Autodesk Fusion 360 part; units mm, degrees
(part 3 of 3)
  line L0 (23, 43.2567) -> (0, 43.2567)
  line L1 (0, 43.2567) -> (0, 32.1215)
  line L2 (0, 32.1215) -> (23, 32.1215)
  line L3 (23, 32.1215) -> (23, 43.2567)
  point P0 (22.9203, 43.2088)
  point P1 (22.8408, 43.161)
  point P2 (22.7615, 43.1132)
  point P3 (22.6824, 43.0656)
  point P4 (22.6036, 43.018)
  point P5 (22.5249, 42.9705)
  point P6 (22.4465, 42.9231)
  point P7 (22.3683, 42.8757)
  point P8 (22.2903, 42.8285)
  point P9 (22.2126, 42.7813)
  point P10 (22.135, 42.7342)
  point P11 (22.0577, 42.6872)
  point P12 (21.9806, 42.6403)
  point P13 (21.9036, 42.5935)
  point P14 (21.827, 42.5468)
  point P15 (21.7505, 42.5001)
  point P16 (21.6742, 42.4536)
  point P17 (21.5981, 42.4071)
  point P18 (21.5223, 42.3607)
  point P19 (21.4467, 42.3144)
  point P20 (21.3713, 42.2682)
  point P21 (21.2961, 42.2221)
  point P22 (21.2211, 42.1761)
  point P23 (21.1463, 42.1302)
  point P24 (21.0717, 42.0844)
  point P25 (20.9973, 42.0386)
  point P26 (20.9232, 41.993)
  point P27 (20.8492, 41.9475)
  point P28 (20.7755, 41.902)
  point P29 (20.702, 41.8567)
  point P30 (20.6287, 41.8115)
  point P31 (20.5556, 41.7663)
  point P32 (20.4827, 41.7213)
  point P33 (20.41, 41.6763)
  point P34 (20.3375, 41.6315)
  point P35 (20.2652, 41.5867)
  point P36 (20.1931, 41.5421)
  point P37 (20.1212, 41.4975)
  point P38 (20.0496, 41.4531)
  point P39 (19.9781, 41.4087)
  point P40 (19.9068, 41.3645)
  point P41 (19.8358, 41.3204)
  point P42 (19.7649, 41.2763)
  point P43 (19.6943, 41.2324)
  point P44 (19.6238, 41.1886)
  point P45 (19.5536, 41.1448)
  point P46 (19.4835, 41.1012)
  point P47 (19.4137, 41.0577)
  point P48 (19.344, 41.0143)
  point P49 (19.2746, 40.971)
  point P50 (19.2054, 40.9278)
  point P51 (19.1363, 40.8848)
  point P52 (19.0674, 40.8418)
  point P53 (18.9988, 40.7989)
  point P54 (18.9303, 40.7562)
  point P55 (18.8621, 40.7135)
  point P56 (18.794, 40.671)
  point P57 (18.7261, 40.6285)
  point P58 (18.6585, 40.5862)
  point P59 (18.591, 40.544)
  point P60 (18.5237, 40.5019)
  point P61 (18.4566, 40.4599)
  point P62 (18.3897, 40.418)
  point P63 (18.323, 40.3763)
  point P64 (18.2565, 40.3346)
  point P65 (18.1901, 40.2931)
  point P66 (18.124, 40.2516)
  point P67 (18.0581, 40.2103)
  point P68 (17.9923, 40.1691)
  point P69 (17.9267, 40.128)
  point P70 (17.8613, 40.0871)
  point P71 (17.7962, 40.0462)
  point P72 (17.7311, 40.0054)
  point P73 (17.6663, 39.9648)
  point P74 (17.6017, 39.9243)
  point P75 (17.5373, 39.8839)
  point P76 (17.473, 39.8436)
  point P77 (17.4089, 39.8034)
  point P78 (17.345, 39.7633)
  point P79 (17.2813, 39.7234)
  point P80 (17.2178, 39.6835)
  point P81 (17.1544, 39.6438)
  point P82 (17.0913, 39.6042)
  point P83 (17.0283, 39.5647)
  point P84 (16.9655, 39.5254)
  point P85 (16.9029, 39.4861)
  point P86 (16.8404, 39.447)
  point P87 (16.7781, 39.408)
  point P88 (16.7161, 39.3691)
  point P89 (16.6541, 39.3303)
  point P90 (16.5924, 39.2916)
  point P91 (16.5309, 39.2531)
  point P92 (16.4695, 39.2146)
  point P93 (16.4083, 39.1763)
  point P94 (16.3472, 39.1381)
  point P95 (16.2864, 39.1)
  point P96 (16.2257, 39.0621)
  point P97 (16.1652, 39.0242)
  point P98 (16.1048, 38.9865)
  point P99 (16.0447, 38.9489)
  point P100 (15.9847, 38.9114)
  point P101 (15.9248, 38.874)
  point P102 (15.8652, 38.8368)
  point P103 (15.8057, 38.7997)
  point P104 (15.7464, 38.7626)
  point P105 (15.6872, 38.7257)
  point P106 (15.6282, 38.689)
  point P107 (15.5694, 38.6523)
  point P108 (15.5107, 38.6158)
  point P109 (15.4522, 38.5793)
  point P110 (15.3939, 38.543)
  point P111 (15.3357, 38.5068)
  point P112 (15.2778, 38.4708)
  point P113 (15.2199, 38.4348)
  point P114 (15.1622, 38.399)
  point P115 (15.1047, 38.3633)
  point P116 (15.0474, 38.3277)
  point P117 (14.9902, 38.2922)
  point P118 (14.9332, 38.2569)
  point P119 (14.8763, 38.2216)
  point P120 (14.8196, 38.1865)
  point P121 (14.763, 38.1515)
  point P122 (14.7066, 38.1167)
  point P123 (14.6504, 38.0819)
  point P124 (14.5943, 38.0473)
  point P125 (14.5384, 38.0127)
  point P126 (14.4826, 37.9783)
  point P127 (14.427, 37.9441)
  point P128 (14.3715, 37.9099)
  point P129 (14.3162, 37.8758)
  point P130 (14.261, 37.8419)
  point P131 (14.206, 37.8081)
  point P132 (14.1511, 37.7744)
  point P133 (14.0964, 37.7408)
  point P134 (14.0419, 37.7074)
  point P135 (13.9875, 37.6741)
  point P136 (13.9332, 37.6408)
  point P137 (13.8791, 37.6077)
  point P138 (13.8251, 37.5748)
  point P139 (13.7713, 37.5419)
  point P140 (13.7176, 37.5092)
  point P141 (13.6641, 37.4765)
  point P142 (13.6107, 37.444)
  point P143 (13.5575, 37.4116)
  point P144 (13.5044, 37.3794)
  point P145 (13.4514, 37.3472)
  point P146 (13.3986, 37.3152)
  point P147 (13.3459, 37.2832)
  point P148 (13.2934, 37.2514)
  point P149 (13.241, 37.2198)
  point P150 (13.1888, 37.1882)
  point P151 (13.1367, 37.1567)
  point P152 (13.0847, 37.1254)
  point P153 (13.0329, 37.0942)
  point P154 (12.9812, 37.0631)
  point P155 (12.9296, 37.0321)
  point P156 (12.8782, 37.0012)
  point P157 (12.8269, 36.9705)
  point P158 (12.7758, 36.9398)
  point P159 (12.7248, 36.9093)
  point P160 (12.6739, 36.8789)
  point P161 (12.6232, 36.8486)
  point P162 (12.5725, 36.8184)
  point P163 (12.5221, 36.7884)
  point P164 (12.4717, 36.7584)
  point P165 (12.4215, 36.7286)
  point P166 (12.3714, 36.6989)
  point P167 (12.3215, 36.6693)
  point P168 (12.2716, 36.6398)
  point P169 (12.2219, 36.6104)
  point P170 (12.1724, 36.5812)
  point P171 (12.1229, 36.5521)
  point P172 (12.0736, 36.523)
  point P173 (12.0244, 36.4941)
  point P174 (11.9753, 36.4653)
  point P175 (11.9264, 36.4366)
  point P176 (11.8776, 36.4081)
  point P177 (11.8289, 36.3796)
  point P178 (11.7803, 36.3513)
  point P179 (11.7319, 36.323)
  point P180 (11.6836, 36.2949)
  point P181 (11.6354, 36.2669)
  point P182 (11.5873, 36.239)
  point P183 (11.5393, 36.2112)
  point P184 (11.4915, 36.1836)
  point P185 (11.4438, 36.156)
  point P186 (11.3962, 36.1286)
  point P187 (11.3487, 36.1012)
  point P188 (11.3013, 36.074)
  point P189 (11.2541, 36.0469)
  point P190 (11.2069, 36.0199)
  point P191 (11.1599, 35.993)
  point P192 (11.113, 35.9662)
  point P193 (11.0662, 35.9396)
  point P194 (11.0196, 35.913)
  point P195 (10.973, 35.8866)
  point P196 (10.9265, 35.8602)
  point P197 (10.8802, 35.834)
  point P198 (10.834, 35.8079)
  point P199 (10.7879, 35.7819)
  point P200 (10.7419, 35.756)
  point P201 (10.696, 35.7302)
  point P202 (10.6502, 35.7045)
  point P203 (10.6046, 35.6789)
  point P204 (10.559, 35.6535)
  point P205 (10.5135, 35.6281)
  point P206 (10.4682, 35.6028)
  point P207 (10.423, 35.5777)
  point P208 (10.3778, 35.5527)
  point P209 (10.3328, 35.5277)
  point P210 (10.2879, 35.5029)
  point P211 (10.2431, 35.4782)
  point P212 (10.1984, 35.4536)
  point P213 (10.1538, 35.4291)
  point P214 (10.1093, 35.4047)
  point P215 (10.0649, 35.3804)
  point P216 (10.0206, 35.3563)
  point P217 (9.9764, 35.3322)
  point P218 (9.9323, 35.3082)
  point P219 (9.8883, 35.2844)
  point P220 (9.8444, 35.2606)
  point P221 (9.8006, 35.2369)
  point P222 (9.7569, 35.2134)
  point P223 (9.7133, 35.19)
  point P224 (9.6698, 35.1666)
  point P225 (9.6264, 35.1434)
  point P226 (9.5831, 35.1202)
  point P227 (9.5399, 35.0972)
  point P228 (9.4968, 35.0743)
  point P229 (9.4538, 35.0515)
  point P230 (9.4109, 35.0288)
  point P231 (9.3681, 35.0061)
  point P232 (9.3253, 34.9836)
  point P233 (9.2827, 34.9612)
  point P234 (9.2402, 34.9389)
  point P235 (9.1977, 34.9167)
  point P236 (9.1553, 34.8946)
  point P237 (9.1131, 34.8726)
  point P238 (9.0709, 34.8507)
  point P239 (9.0288, 34.8289)
  point P240 (8.9868, 34.8072)
  point P241 (8.9449, 34.7856)
  point P242 (8.9031, 34.7641)
  point P243 (8.8614, 34.7427)
  point P244 (8.8197, 34.7214)
  point P245 (8.7782, 34.7002)
  point P246 (8.7367, 34.6791)
  point P247 (8.6953, 34.6581)
  point P248 (8.6541, 34.6373)
  point P249 (8.6128, 34.6165)
  point P250 (8.5717, 34.5958)
  point P251 (8.5307, 34.5752)
  point P252 (8.4897, 34.5547)
  point P253 (8.4489, 34.5343)
  point P254 (8.4081, 34.514)
  point P255 (8.3674, 34.4937)
  point P256 (8.3268, 34.4736)
  point P257 (8.2862, 34.4536)
  point P258 (8.2458, 34.4337)
  point P259 (8.2054, 34.4139)
  point P260 (8.1651, 34.3942)
  point P261 (8.1249, 34.3746)
  point P262 (8.0848, 34.355)
  point P263 (8.0447, 34.3356)
  point P264 (8.0048, 34.3163)
  point P265 (7.9649, 34.297)
  point P266 (7.925, 34.2779)
  point P267 (7.8853, 34.2588)
  point P268 (7.8456, 34.2399)
  point P269 (7.806, 34.221)
  point P270 (7.7665, 34.2023)
  point P271 (7.7271, 34.1836)
  point P272 (7.6877, 34.165)
  point P273 (7.6485, 34.1466)
  point P274 (7.6093, 34.1282)
  point P275 (7.5701, 34.1099)
  point P276 (7.5311, 34.0917)
  point P277 (7.4921, 34.0736)
  point P278 (7.4531, 34.0556)
  point P279 (7.4143, 34.0377)
  point P280 (7.3755, 34.0198)
  point P281 (7.3368, 34.0021)
  point P282 (7.2982, 33.9845)
  point P283 (7.2596, 33.9669)
  point P284 (7.2211, 33.9495)
  point P285 (7.1827, 33.9321)
  point P286 (7.1444, 33.9148)
  point P287 (7.1061, 33.8977)
  point P288 (7.0679, 33.8806)
  point P289 (7.0297, 33.8636)
  point P290 (6.9917, 33.8467)
  point P291 (6.9536, 33.8299)
  point P292 (6.9157, 33.8131)
  point P293 (6.8778, 33.7965)
  point P294 (6.84, 33.78)
  point P295 (6.8023, 33.7635)
  point P296 (6.7646, 33.7472)
  point P297 (6.727, 33.7309)
  point P298 (6.6894, 33.7147)
  point P299 (6.6519, 33.6986)
  point P300 (6.6145, 33.6826)
  point P301 (6.5771, 33.6667)
  point P302 (6.5398, 33.6509)
  point P303 (6.5026, 33.6351)
  point P304 (6.4654, 33.6195)
  point P305 (6.4283, 33.6039)
  point P306 (6.3913, 33.5885)
  point P307 (6.3543, 33.5731)
  point P308 (6.3173, 33.5578)
  point P309 (6.2805, 33.5426)
  point P310 (6.2437, 33.5274)
  point P311 (6.2069, 33.5124)
  point P312 (6.1702, 33.4975)
  point P313 (6.1336, 33.4826)
  point P314 (6.097, 33.4678)
  point P315 (6.0605, 33.4532)
  point P316 (6.024, 33.4386)
  point P317 (5.9876, 33.424)
  point P318 (5.9513, 33.4096)
  point P319 (5.915, 33.3953)
  point P320 (5.8788, 33.381)
  point P321 (5.8426, 33.3669)
  point P322 (5.8064, 33.3528)
  point P323 (5.7704, 33.3388)
  point P324 (5.7344, 33.3249)
  point P325 (5.6984, 33.311)
  point P326 (5.6625, 33.2973)
  point P327 (5.6266, 33.2837)
  point P328 (5.5908, 33.2701)
  point P329 (5.5551, 33.2566)
  point P330 (5.5194, 33.2432)
  point P331 (5.4837, 33.2299)
  point P332 (5.4481, 33.2166)
  point P333 (5.4126, 33.2035)
  point P334 (5.3771, 33.1904)
  point P335 (5.3417, 33.1774)
  point P336 (5.3063, 33.1645)
  point P337 (5.2709, 33.1517)
  point P338 (5.2356, 33.139)
  point P339 (5.2004, 33.1263)
  point P340 (5.1652, 33.1138)
  point P341 (5.13, 33.1013)
  point P342 (5.0949, 33.0889)
  point P343 (5.0599, 33.0766)
  point P344 (5.0249, 33.0643)
  point P345 (4.9899, 33.0522)
  point P346 (4.955, 33.0401)
  point P347 (4.9201, 33.0281)
  point P348 (4.8853, 33.0162)
  point P349 (4.8505, 33.0044)
  point P350 (4.8158, 32.9927)
  point P351 (4.7811, 32.981)
  point P352 (4.7465, 32.9694)
  point P353 (4.7119, 32.9579)
  point P354 (4.6773, 32.9465)
  point P355 (4.6428, 32.9352)
  point P356 (4.6084, 32.9239)
  point P357 (4.5739, 32.9127)
  point P358 (4.5396, 32.9016)
  point P359 (4.5052, 32.8906)
  point P360 (4.4709, 32.8797)
  point P361 (4.4367, 32.8689)
  point P362 (4.4025, 32.8581)
  point P363 (4.3683, 32.8474)
  point P364 (4.3341, 32.8368)
  point P365 (4.3001, 32.8262)
  point P366 (4.266, 32.8158)
  point P367 (4.232, 32.8054)
  point P368 (4.198, 32.7951)
  point P369 (4.1641, 32.7849)
  point P370 (4.1302, 32.7748)
  point P371 (4.0963, 32.7647)
  point P372 (4.0625, 32.7548)
  point P373 (4.0287, 32.7449)
  point P374 (3.995, 32.7351)
  point P375 (3.9612, 32.7253)
  point P376 (3.9276, 32.7157)
  point P377 (3.8939, 32.7061)
  point P378 (3.8603, 32.6966)
  point P379 (3.8268, 32.6872)
  point P380 (3.7932, 32.6778)
  point P381 (3.7597, 32.6686)
  point P382 (3.7263, 32.6594)
  point P383 (3.6928, 32.6503)
  point P384 (3.6595, 32.6413)
  point P385 (3.6261, 32.6323)
  point P386 (3.5928, 32.6235)
  point P387 (3.5595, 32.6147)
  point P388 (3.5262, 32.6059)
  point P389 (3.493, 32.5973)
  point P390 (3.4598, 32.5888)
  point P391 (3.4266, 32.5803)
  point P392 (3.3935, 32.5719)
  point P393 (3.3604, 32.5636)
  point P394 (3.3273, 32.5553)
  point P395 (3.2943, 32.5471)
  point P396 (3.2613, 32.5391)
  point P397 (3.2283, 32.531)
  point P398 (3.1954, 32.5231)
  point P399 (3.1624, 32.5152)
  point P400 (3.1295, 32.5075)
  point P401 (3.0967, 32.4998)
  point P402 (3.0638, 32.4921)
  point P403 (3.031, 32.4846)
  point P404 (2.9983, 32.4771)
  point P405 (2.9655, 32.4697)
  point P406 (2.9328, 32.4624)
  point P407 (2.9001, 32.4552)
  point P408 (2.8674, 32.448)
  point P409 (2.8348, 32.4409)
  point P410 (2.8022, 32.4339)
  point P411 (2.7696, 32.427)
  point P412 (2.737, 32.4202)
  point P413 (2.7045, 32.4134)
  point P414 (2.672, 32.4067)
  point P415 (2.6395, 32.4001)
  point P416 (2.607, 32.3935)
  point P417 (2.5746, 32.387)
  point P418 (2.5421, 32.3807)
  point P419 (2.5098, 32.3743)
  point P420 (2.4774, 32.3681)
  point P421 (2.445, 32.3619)
  point P422 (2.4127, 32.3559)
  point P423 (2.3804, 32.3499)
  point P424 (2.3481, 32.3439)
  point P425 (2.3159, 32.3381)
  point P426 (2.2836, 32.3323)
  point P427 (2.2514, 32.3266)
  point P428 (2.2192, 32.321)
  point P429 (2.187, 32.3154)
  point P430 (2.1549, 32.31)
  point P431 (2.1227, 32.3046)
  point P432 (2.0906, 32.2993)
  point P433 (2.0585, 32.294)
  point P434 (2.0265, 32.2889)
  point P435 (1.9944, 32.2838)
  point P436 (1.9624, 32.2788)
  point P437 (1.9303, 32.2739)
  point P438 (1.8983, 32.269)
  point P439 (1.8663, 32.2642)
  point P440 (1.8344, 32.2595)
  point P441 (1.8024, 32.2549)
  point P442 (1.7705, 32.2504)
  point P443 (1.7386, 32.2459)
  point P444 (1.7067, 32.2415)
  point P445 (1.6748, 32.2372)
  point P446 (1.6429, 32.233)
  point P447 (1.6111, 32.2288)
  point P448 (1.5792, 32.2248)
  point P449 (1.5474, 32.2208)
  point P450 (1.5156, 32.2168)
  point P451 (1.4838, 32.213)
  point P452 (1.452, 32.2092)
  point P453 (1.4202, 32.2055)
  point P454 (1.3885, 32.2019)
  point P455 (1.3567, 32.1984)
  point P456 (1.325, 32.1949)
  point P457 (1.2933, 32.1916)
  point P458 (1.2616, 32.1883)
  point P459 (1.2299, 32.185)
  point P460 (1.1982, 32.1819)
  point P461 (1.1665, 32.1788)
  point P462 (1.1349, 32.1758)
  point P463 (1.1032, 32.1729)
  point P464 (1.0716, 32.1701)
  point P465 (1.04, 32.1674)
  point P466 (1.0083, 32.1647)
  point P467 (0.9767, 32.1621)
  point P468 (0.9451, 32.1596)
  point P469 (0.9135, 32.1571)
  point P470 (0.882, 32.1548)
  point P471 (0.8504, 32.1525)
  point P472 (0.8188, 32.1503)
  point P473 (0.7873, 32.1482)
  point P474 (0.7557, 32.1462)
  point P475 (0.7242, 32.1442)
  point P476 (0.6926, 32.1423)
  point P477 (0.6611, 32.1405)
  point P478 (0.6296, 32.1388)
  point P479 (0.5981, 32.1372)
  point P480 (0.5666, 32.1356)
  point P481 (0.535, 32.1341)
  point P482 (0.5035, 32.1327)
  point P483 (0.472, 32.1314)
  point P484 (0.4406, 32.1302)
  point P485 (0.4091, 32.129)
  point P486 (0.3776, 32.128)
  point P487 (0.3461, 32.127)
  point P488 (0.3146, 32.1261)
  point P489 (0.2832, 32.1253)
  point P490 (0.2517, 32.1245)
  point P491 (0.2202, 32.1238)
  point P492 (0.1888, 32.1233)
  point P493 (0.1573, 32.1228)
  point P494 (0.1258, 32.1223)
  point P495 (0.0944, 32.122)
  point P496 (0.0629, 32.1218)
  point P497 (0.0315, 32.1216)
  constraint horizontal L0
  constraint vertical L1
  constraint horizontal L2
  constraint vertical L3
revolve "回転1" add sketch "スケッチ1" angle 360 about axis through (0, 43.2567, 0) along (0, -1, 0) contours S0 L0 L1
sketch "スケッチ4" plane through (0, 0, 0) normal (0, 0, 1) x (1, 0, 0)
  circle A0 centre (0, 0) radius 23
  dimension "d3" = 46
  constraint coincident A0.centre origin
  measures "d3" diameter of A0
move_body "移動1" bodies 1 to x (1, 0, 0) y (0, 0, 1) z (0, -1, 0) at (0, 9.1215, -55.1215)
move_body "移動2" bodies 1 to x (1, 0, 0) y (0, -1, 0) z (0, 0, -1) at (0, -27.757, -46)
move_body "移動3" bodies 1 to x (1, 0, 0) y (0, 1, 0) z (0, 0, 1) at (0, 36.8785, 34.1352)
